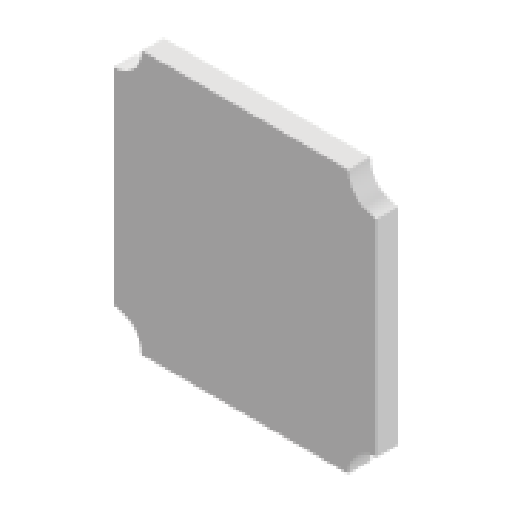
# Autodesk Inventor part: whiteLEDArray
Saved by Autodesk Inventor 2026.1 (Build 301233000, 233)
## iProperties
Created: 2026-03-05
Part Number: whiteLEDArray
Material: Generic
Document SubType Name: Modeling
Designer: aleja
Density: 1 g/cm^3
Appearance: Default
Author: aleja
Autodesk Inventor part; units mm, degrees
ref_plane "YZ Plane" through (0, 0, 0) normal (1, 0, 0) x (0, 1, 0)
ref_plane "XZ Plane" through (0, 0, 0) normal (0, 1, 0) x (-1, 0, 0)
ref_plane "XY Plane" through (0, 0, 0) normal (0, 0, 1) x (1, 0, 0)
sketch "Sketch1" plane through (0, 0, 0) normal (0, 1, 0) x (-1, 0, 0)
  line L0 (13.25, -13.25) -> (-13.25, -13.25)
  line L1 (-13.25, -13.25) -> (-13.25, 13.25)
  line L2 (-13.25, 13.25) -> (13.25, 13.25)
  line L3 (13.25, 13.25) -> (13.25, -13.25)
  line L4 (13.25, -13.25) -> (-13.25, 13.25) construction
  line L5 (-13.25, -13.25) -> (13.25, 13.25) construction
  circle A0 centre (13.25, 13.25) radius 2.6
  line L6 (0, 0) -> (0, 4.9748) construction
  line L7 (0, 0) -> (-3.9758, 0) construction
  circle A1 centre (-13.25, 13.25) radius 2.6
  line L8 (0, 0) -> (3.9758, 0) construction
  circle A2 centre (13.25, -13.25) radius 2.6
  circle A3 centre (-13.25, -13.25) radius 2.6
  point P0 (-13.25, -10.65)
  point P1 (-10.65, -13.25)
  point P2 (10.65, -13.25)
  point P3 (13.25, -10.65)
  point P4 (13.25, 10.65)
  point P5 (10.65, 13.25)
  point P6 (-10.65, 13.25)
  point P7 (-13.25, 10.65)
  dimension "d0" = 26.5
  dimension "d1" = 26.5
  dimension "d2" = 5.2
  constraints: 18 end point, 4 centre point, 4 symmetric about line, 2 horizontal, 2 midpoint, 2 parallel, 1 coincident, 1 perpendicular, 1 vertical, 3 other
  measures "d0" distance of L1.end L2.end
  measures "d1" distance of L0.end L1.end
  measures "d2" diameter of A0
extrude "Extrusion1" add sketch "Sketch1" along normal blind 2 contours A3 L1 A1 L2 A0 L3 A2 L0
sketch "Sketch2" plane through (0, 0, 0) normal (0, -1, 0) x (1, 0, 0)
  line L0 (-9, 7) -> (-7, 7)
  line L1 (-7, 7) -> (-7, 9)
  line L2 (-7, 9) -> (-9, 9)
  line L3 (-9, 9) -> (-9, 7)
  line L4 (-9, 7) -> (-7, 9) construction
  line L5 (-7, 7) -> (-9, 9) construction
  line L6 (-3.8, 9) -> (-5.8, 9)
  line L7 (-3.8, 7) -> (-3.8, 9)
  line L8 (-5.8, 9) -> (-5.8, 7)
  line L9 (-5.8, 7) -> (-3.8, 7)
  line L10 (-0.6, 9) -> (-2.6, 9)
  line L11 (-0.6, 7) -> (-0.6, 9)
  line L12 (-2.6, 9) -> (-2.6, 7)
  line L13 (-2.6, 7) -> (-0.6, 7)
  line L14 (2.6, 9) -> (0.6, 9)
  line L15 (2.6, 7) -> (2.6, 9)
  line L16 (0.6, 9) -> (0.6, 7)
  line L17 (0.6, 7) -> (2.6, 7)
  line L18 (5.8, 9) -> (3.8, 9)
  line L19 (5.8, 7) -> (5.8, 9)
  line L20 (3.8, 9) -> (3.8, 7)
  line L21 (3.8, 7) -> (5.8, 7)
  line L22 (9, 9) -> (7, 9)
  line L23 (9, 7) -> (9, 9)
  line L24 (7, 9) -> (7, 7)
  line L25 (7, 7) -> (9, 7)
  line L26 (-7, 5.8) -> (-9, 5.8)
  line L27 (-7, 3.8) -> (-7, 5.8)
  line L28 (-9, 5.8) -> (-9, 3.8)
  line L29 (-9, 3.8) -> (-7, 3.8)
  line L30 (-3.8, 5.8) -> (-5.8, 5.8)
  line L31 (-3.8, 3.8) -> (-3.8, 5.8)
  line L32 (-5.8, 5.8) -> (-5.8, 3.8)
  line L33 (-5.8, 3.8) -> (-3.8, 3.8)
  line L34 (-0.6, 5.8) -> (-2.6, 5.8)
  line L35 (-0.6, 3.8) -> (-0.6, 5.8)
  line L36 (-2.6, 5.8) -> (-2.6, 3.8)
  line L37 (-2.6, 3.8) -> (-0.6, 3.8)
  line L38 (2.6, 5.8) -> (0.6, 5.8)
  line L39 (2.6, 3.8) -> (2.6, 5.8)
  line L40 (0.6, 5.8) -> (0.6, 3.8)
  line L41 (0.6, 3.8) -> (2.6, 3.8)
  line L42 (5.8, 5.8) -> (3.8, 5.8)
  line L43 (5.8, 3.8) -> (5.8, 5.8)
  line L44 (3.8, 5.8) -> (3.8, 3.8)
  line L45 (3.8, 3.8) -> (5.8, 3.8)
  line L46 (9, 5.8) -> (7, 5.8)
  line L47 (9, 3.8) -> (9, 5.8)
  line L48 (7, 5.8) -> (7, 3.8)
  line L49 (7, 3.8) -> (9, 3.8)
  line L50 (-7, 2.6) -> (-9, 2.6)
  line L51 (-7, 0.6) -> (-7, 2.6)
  line L52 (-9, 2.6) -> (-9, 0.6)
  line L53 (-9, 0.6) -> (-7, 0.6)
  line L54 (-3.8, 2.6) -> (-5.8, 2.6)
  line L55 (-3.8, 0.6) -> (-3.8, 2.6)
  line L56 (-5.8, 2.6) -> (-5.8, 0.6)
  line L57 (-5.8, 0.6) -> (-3.8, 0.6)
  line L58 (-0.6, 2.6) -> (-2.6, 2.6)
  line L59 (-0.6, 0.6) -> (-0.6, 2.6)
  line L60 (-2.6, 2.6) -> (-2.6, 0.6)
  line L61 (-2.6, 0.6) -> (-0.6, 0.6)
  line L62 (2.6, 2.6) -> (0.6, 2.6)
  line L63 (2.6, 0.6) -> (2.6, 2.6)
  line L64 (0.6, 2.6) -> (0.6, 0.6)
  line L65 (0.6, 0.6) -> (2.6, 0.6)
  line L66 (5.8, 2.6) -> (3.8, 2.6)
  line L67 (5.8, 0.6) -> (5.8, 2.6)
  line L68 (3.8, 2.6) -> (3.8, 0.6)
  line L69 (3.8, 0.6) -> (5.8, 0.6)
  line L70 (9, 2.6) -> (7, 2.6)
  line L71 (9, 0.6) -> (9, 2.6)
  line L72 (7, 2.6) -> (7, 0.6)
  line L73 (7, 0.6) -> (9, 0.6)
  line L74 (-7, -0.6) -> (-9, -0.6)
  line L75 (-7, -2.6) -> (-7, -0.6)
  line L76 (-9, -0.6) -> (-9, -2.6)
  line L77 (-9, -2.6) -> (-7, -2.6)
  line L78 (-3.8, -0.6) -> (-5.8, -0.6)
  line L79 (-3.8, -2.6) -> (-3.8, -0.6)
  line L80 (-5.8, -0.6) -> (-5.8, -2.6)
  line L81 (-5.8, -2.6) -> (-3.8, -2.6)
  line L82 (-0.6, -0.6) -> (-2.6, -0.6)
  line L83 (-0.6, -2.6) -> (-0.6, -0.6)
  line L84 (-2.6, -0.6) -> (-2.6, -2.6)
  line L85 (-2.6, -2.6) -> (-0.6, -2.6)
  line L86 (2.6, -0.6) -> (0.6, -0.6)
  line L87 (2.6, -2.6) -> (2.6, -0.6)
  line L88 (0.6, -0.6) -> (0.6, -2.6)
  line L89 (0.6, -2.6) -> (2.6, -2.6)
  line L90 (5.8, -0.6) -> (3.8, -0.6)
  line L91 (5.8, -2.6) -> (5.8, -0.6)
  line L92 (3.8, -0.6) -> (3.8, -2.6)
  line L93 (3.8, -2.6) -> (5.8, -2.6)
  line L94 (9, -0.6) -> (7, -0.6)
  line L95 (9, -2.6) -> (9, -0.6)
  line L96 (7, -0.6) -> (7, -2.6)
  line L97 (7, -2.6) -> (9, -2.6)
  line L98 (-7, -3.8) -> (-9, -3.8)
  line L99 (-7, -5.8) -> (-7, -3.8)
  line L100 (-9, -3.8) -> (-9, -5.8)
  line L101 (-9, -5.8) -> (-7, -5.8)
  line L102 (-3.8, -3.8) -> (-5.8, -3.8)
  line L103 (-3.8, -5.8) -> (-3.8, -3.8)
  line L104 (-5.8, -3.8) -> (-5.8, -5.8)
  line L105 (-5.8, -5.8) -> (-3.8, -5.8)
  line L106 (-0.6, -3.8) -> (-2.6, -3.8)
  line L107 (-0.6, -5.8) -> (-0.6, -3.8)
  line L108 (-2.6, -3.8) -> (-2.6, -5.8)
  line L109 (-2.6, -5.8) -> (-0.6, -5.8)
  line L110 (2.6, -3.8) -> (0.6, -3.8)
  line L111 (2.6, -5.8) -> (2.6, -3.8)
  line L112 (0.6, -3.8) -> (0.6, -5.8)
  line L113 (0.6, -5.8) -> (2.6, -5.8)
  line L114 (5.8, -3.8) -> (3.8, -3.8)
  line L115 (5.8, -5.8) -> (5.8, -3.8)
  line L116 (3.8, -3.8) -> (3.8, -5.8)
  line L117 (3.8, -5.8) -> (5.8, -5.8)
  line L118 (9, -3.8) -> (7, -3.8)
  line L119 (9, -5.8) -> (9, -3.8)
  line L120 (7, -3.8) -> (7, -5.8)
  line L121 (7, -5.8) -> (9, -5.8)
  line L122 (-7, -7) -> (-9, -7)
  line L123 (-7, -9) -> (-7, -7)
  line L124 (-9, -7) -> (-9, -9)
  line L125 (-9, -9) -> (-7, -9)
  line L126 (-3.8, -7) -> (-5.8, -7)
  line L127 (-3.8, -9) -> (-3.8, -7)
  line L128 (-5.8, -7) -> (-5.8, -9)
  line L129 (-5.8, -9) -> (-3.8, -9)
  line L130 (-0.6, -7) -> (-2.6, -7)
  line L131 (-0.6, -9) -> (-0.6, -7)
  line L132 (-2.6, -7) -> (-2.6, -9)
  line L133 (-2.6, -9) -> (-0.6, -9)
  line L134 (2.6, -7) -> (0.6, -7)
  line L135 (2.6, -9) -> (2.6, -7)
  line L136 (0.6, -7) -> (0.6, -9)
  line L137 (0.6, -9) -> (2.6, -9)
  line L138 (5.8, -7) -> (3.8, -7)
  line L139 (5.8, -9) -> (5.8, -7)
  line L140 (3.8, -7) -> (3.8, -9)
  line L141 (3.8, -9) -> (5.8, -9)
  line L142 (9, -7) -> (7, -7)
  line L143 (9, -9) -> (9, -7)
  line L144 (7, -7) -> (7, -9)
  line L145 (7, -9) -> (9, -9)
  point P0 (0, 0)
  point P1 (-8, 8)
  dimension "d5" = 2
  dimension "d6" = 2
  dimension "d9" = 3.2
  dimension "d12" = 3.2
  dimension "d15" = 8
  dimension "d16" = 8
  constraints: 292 end point, 2 collinear, 2 horizontal, 2 midpoint, 2 parallel, 1 perpendicular, 1 vertical, 278 other
  measures "d5" distance of L2.end L1.end
  measures "d6" distance of L1.end L0.end
  measures "d9" distance of L1.end L6.start
  measures "d12" distance of L1.end L26.start
  measures "d15" horizontal distance of point (0, 0) point (-8, 8)
  measures "d16" horizontal distance of point (-8, 8) point (0, 0)
extrude "Extrusion2" add sketch "Sketch2" along normal blind 1
equation "\"d1\" = d0"
equation "\"d5\" = d6"
equation "\"d9\" = d12"
body "Solid1"
